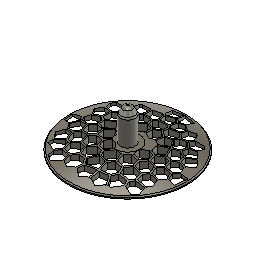
CD Labeler v6 (Autodesk Fusion 360 design; units mm, degrees)
Autodesk Fusion 360 part; units mm, degrees
sketch "Sketch1" plane through (0, 0, 0) normal (0, 0, 1) x (1, 0, 0)
  line L0 (0, 0) -> (-60, 0)
  line L1 (0, 40) -> (-7.4, 40)
  line L2 (-7.4, 40) -> (-7.4, 7.5)
  line L3 (-7.4, 7.5) -> (-12.4, 7.5)
  line L4 (-60, 0) -> (-60, 2)
  spline S0 degree 5 poles (-60, 2) (-58.1311, 2.342) (-54.3892, 3.0118) (-48.7641, 3.9741) (-41.2378, 5.166) (-31.765, 6.4302) (-24.1021, 7.147) (-18.2833, 7.4358) (-14.3673, 7.5) (-12.4, 7.5) knots 0 0 0 0 0 0 0.2 0.4 0.6 0.8 1 1 1 1 1 1
  line L5 (-17.4, 7.5) -> (-7.4, 7.5)
  line L6 (0, 40) -> (0, 0)
  dimension "d5" = 60
  dimension "d6" = 40
  dimension "d7" = 7.5
  dimension "d8" = 5
  dimension "d9" = 7.4
  dimension "d10" = 2
  constraint coincident L0.start L6.end
  constraint horizontal L0
  constraint perpendicular L1 L2
  constraint perpendicular L2 L3
  constraint vertical L0.start L1.start
  constraint perpendicular L0 L4
  constraint midpoint L3.end L5
  constraint coincident L2.end L3.start
  measures "d5" distance of L0.start L0.end
  measures "d6" distance of L0.start L1.start
  measures "d7" distance of L0 L3
  measures "d8" distance of L2.end L3.end
  measures "d9" distance of L0.start L2
  measures "d10" distance of L0.end L4.end
revolve "Revolve1" add sketch "Sketch1" angle 360 about axis through (0, 40, 0) along (0, -1, 0)
chamfer "Chamfer1" distance 4 angle 60 1 edges at (-6.8992, 40, 2.676) measured on face at (-1.4729, 40, 2.6203)
fillet "Fillet1" radius 4 2 edges at (-3.1699, 40, -1.2295) (-6.8992, 33.0718, 2.676)
chamfer "Chamfer2" distance 1 angle 45 1 edges at (-55.9396, 2, 21.6969) measured on face at (-50.8568, 3.2274, -15.1547)
sketch "Voronoi" plane through (0, 0, 0) normal (0, -1, 0) x (1, 0, 0)
  circle A0 centre (0, 0) radius 60
  line L0 (-27.9065, 13.1696) -> (-34.9281, 12.0421)
  line L1 (-34.9281, 12.0421) -> (-38.6848, 16.0627)
  line L2 (-38.6848, 16.0627) -> (-35.8746, 24.3668)
  line L3 (-35.8746, 24.3668) -> (-32.044, 25.7826)
  line L4 (-32.044, 25.7826) -> (-26.0586, 21.4152)
  line L5 (-26.0586, 21.4152) -> (-27.9065, 13.1696)
  line L6 (10.5368, 0.5792) -> (4.8128, -2.3641)
  line L7 (4.8128, -2.3641) -> (0.9891, -1.0588)
  line L8 (0.9891, -1.0588) -> (-2.1672, 4.4874)
  line L9 (-2.1672, 4.4874) -> (1.2988, 10.7375)
  line L10 (1.2988, 10.7375) -> (7.2211, 11.6685)
  line L11 (7.2211, 11.6685) -> (11.5672, 7.4823)
  line L12 (11.5672, 7.4823) -> (10.5368, 0.5792)
  line L13 (-35.0108, -24.4064) -> (-34.1777, -32.4462)
  line L14 (-34.1777, -32.4462) -> (-44.9989, -34.043)
  line L15 (-44.9989, -34.043) -> (-47.8212, -30.2156)
  line L16 (-47.8212, -30.2156) -> (-46.0411, -24.2468)
  line L17 (-46.0411, -24.2468) -> (-38.1193, -22.0129)
  line L18 (-38.1193, -22.0129) -> (-35.0108, -24.4064)
  line L19 (-19.5879, 24.2667) -> (-25.0625, 22.7039)
  line L20 (-25.0625, 22.7039) -> (-31.0479, 27.0713)
  line L21 (-31.0479, 27.0713) -> (-29.3019, 34.4485)
  line L22 (-29.3019, 34.4485) -> (-21.5865, 36.5994)
  line L23 (-21.5865, 36.5994) -> (-17.0949, 32.1475)
  line L24 (-17.0949, 32.1475) -> (-19.5879, 24.2667)
  line L25 (-46.2354, -10.1125) -> (-38.6533, -12.4637)
  line L26 (-38.6533, -12.4637) -> (-38.56, -20.628)
  line L27 (-38.56, -20.628) -> (-46.4818, -22.862)
  line L28 (-46.4818, -22.862) -> (-50.7842, -17.082)
  line L29 (-50.7842, -17.082) -> (-46.2354, -10.1125)
  line L30 (-8.096, -27.9757) -> (-9.18, -32.5512)
  line L31 (-9.18, -32.5512) -> (-18.5579, -34.2016)
  line L32 (-18.5579, -34.2016) -> (-20.6222, -32.1222)
  line L33 (-20.6222, -32.1222) -> (-19.5242, -22.5311)
  line L34 (-19.5242, -22.5311) -> (-13.2488, -21.94)
  line L35 (-13.2488, -21.94) -> (-8.096, -27.9757)
  line L36 (39.3425, 0.2337) -> (45.9107, 0.9874)
  line L37 (45.9107, 0.9874) -> (49.7447, -4.1853)
  line L38 (49.7447, -4.1853) -> (47.1146, -9.6574)
  line L39 (47.1146, -9.6574) -> (41.0309, -11.0528)
  line L40 (41.0309, -11.0528) -> (36.8887, -6.9194)
  line L41 (36.8887, -6.9194) -> (39.3425, 0.2337)
  line L42 (-18.027, -5.9471) -> (-24.1755, -13.3608)
  line L43 (-24.1755, -13.3608) -> (-32.371, -8.4307)
  line L44 (-32.371, -8.4307) -> (-31.6276, -3.0621)
  line L45 (-31.6276, -3.0621) -> (-24.5907, -0.2592)
  line L46 (-24.5907, -0.2592) -> (-18.027, -5.9471)
  line L47 (10.7696, 22.7391) -> (6.3027, 27.2437)
  line L48 (6.3027, 27.2437) -> (8.1302, 35.9137)
  line L49 (8.1302, 35.9137) -> (8.6268, 36.3055)
  line L50 (8.6268, 36.3055) -> (17.3076, 34.8942)
  line L51 (17.3076, 34.8942) -> (20.1346, 29.6995)
  line L52 (20.1346, 29.6995) -> (17.7876, 23.9489)
  line L53 (17.7876, 23.9489) -> (10.7696, 22.7391)
  line L54 (-11.0886, 4.3113) -> (-15.7382, -4.7739)
  line L55 (-15.7382, -4.7739) -> (-17.0875, -4.8798)
  line L56 (-17.0875, -4.8798) -> (-23.6512, 0.8081)
  line L57 (-23.6512, 0.8081) -> (-22.375, 7.5716)
  line L58 (-22.375, 7.5716) -> (-15.122, 9.0483)
  line L59 (-15.122, 9.0483) -> (-11.0886, 4.3113)
  line L60 (33.8324, -27.9238) -> (33.0464, -21.9044)
  line L61 (33.0464, -21.9044) -> (39.3933, -18.8795)
  line L62 (39.3933, -18.8795) -> (45.5831, -24.6473)
  line L63 (45.5831, -24.6473) -> (39.9794, -30.3799)
  line L64 (39.9794, -30.3799) -> (33.8324, -27.9238)
  line L65 (-6.1734, 20.3155) -> (-12.2476, 18.5647)
  line L66 (-12.2476, 18.5647) -> (-18.0321, 23.7761)
  line L67 (-18.0321, 23.7761) -> (-15.5391, 31.657)
  line L68 (-15.5391, 31.657) -> (-9.0862, 32.5632)
  line L69 (-9.0862, 32.5632) -> (-4.1809, 24.8404)
  line L70 (-4.1809, 24.8404) -> (-6.1734, 20.3155)
  line L71 (-9.34, 34.3958) -> (-15.793, 33.4895)
  line L72 (-15.793, 33.4895) -> (-20.2846, 37.9414)
  line L73 (-20.2846, 37.9414) -> (-19.1442, 45.1176)
  line L74 (-19.1442, 45.1176) -> (-13.5017, 48.1808)
  line L75 (-13.5017, 48.1808) -> (-7.4331, 45.104)
  line L76 (-7.4331, 45.104) -> (-6.1591, 39.3578)
  line L77 (-6.1591, 39.3578) -> (-9.34, 34.3958)
  line L78 (12.2231, 0.3468) -> (13.2535, 7.25)
  line L79 (13.2535, 7.25) -> (20.8866, 9.2558)
  line L80 (20.8866, 9.2558) -> (25.2818, 4.1153)
  line L81 (25.2818, 4.1153) -> (23.592, -1.8074)
  line L82 (23.592, -1.8074) -> (18.3034, -3.8239)
  line L83 (18.3034, -3.8239) -> (12.2231, 0.3468)
  line L84 (21.6213, 30.6504) -> (18.7944, 35.8452)
  line L85 (18.7944, 35.8452) -> (23.926, 44.059)
  line L86 (23.926, 44.059) -> (26.7774, 44.2439)
  line L87 (26.7774, 44.2439) -> (32.4218, 36.8622)
  line L88 (32.4218, 36.8622) -> (30.8724, 31.3991)
  line L89 (30.8724, 31.3991) -> (21.6213, 30.6504)
  line L90 (5.4069, -28.6869) -> (5.7475, -34.199)
  line L91 (5.7475, -34.199) -> (3.4929, -36.7027)
  line L92 (3.4929, -36.7027) -> (-5.3646, -36.1946)
  line L93 (-5.3646, -36.1946) -> (-7.566, -32.9035)
  line L94 (-7.566, -32.9035) -> (-6.482, -28.3281)
  line L95 (-6.482, -28.3281) -> (0.1282, -25.3112)
  line L96 (0.1282, -25.3112) -> (5.4069, -28.6869)
  line L97 (-19.9419, -35.5296) -> (-20.3626, -43.7583)
  line L98 (-20.3626, -43.7583) -> (-21.5377, -44.6998)
  line L99 (-21.5377, -44.6998) -> (-30.0108, -44.8241)
  line L100 (-30.0108, -44.8241) -> (-31.5242, -43.6638)
  line L101 (-31.5242, -43.6638) -> (-31.8434, -34.2746)
  line L102 (-31.8434, -34.2746) -> (-22.0062, -33.4501)
  line L103 (-22.0062, -33.4501) -> (-19.9419, -35.5296)
  line L104 (20.2503, -26.6016) -> (26.1962, -18.8729)
  line L105 (26.1962, -18.8729) -> (31.4796, -22.0469)
  line L106 (31.4796, -22.0469) -> (32.2655, -28.0663)
  line L107 (32.2655, -28.0663) -> (27.2411, -32.7623)
  line L108 (27.2411, -32.7623) -> (21.77, -31.0504)
  line L109 (21.77, -31.0504) -> (20.2503, -26.6016)
  line L110 (-8.9484, -12.5065) -> (-13.447, -20.2206)
  line L111 (-13.447, -20.2206) -> (-19.7224, -20.8116)
  line L112 (-19.7224, -20.8116) -> (-22.4798, -18.4615)
  line L113 (-22.4798, -18.4615) -> (-23.073, -14.1926)
  line L114 (-23.073, -14.1926) -> (-16.9244, -6.779)
  line L115 (-16.9244, -6.779) -> (-15.5751, -6.6731)
  line L116 (-15.5751, -6.6731) -> (-9.2991, -11.2456)
  line L117 (-9.2991, -11.2456) -> (-8.9484, -12.5065)
  line L118 (6.6615, 37.7021) -> (-4.4548, 39.7887)
  line L119 (-4.4548, 39.7887) -> (-5.7288, 45.5349)
  line L120 (-5.7288, 45.5349) -> (1.4543, 51.1494)
  line L121 (1.4543, 51.1494) -> (7.689, 46.826)
  line L122 (7.689, 46.826) -> (7.1581, 38.0939)
  line L123 (7.1581, 38.0939) -> (6.6615, 37.7021)
  line L124 (25.1249, -2.252) -> (26.8147, 3.6707)
  line L125 (26.8147, 3.6707) -> (34.0171, 5.2501)
  line L126 (34.0171, 5.2501) -> (37.9277, 0.7189)
  line L127 (37.9277, 0.7189) -> (35.4738, -6.4342)
  line L128 (35.4738, -6.4342) -> (30.5831, -7.2276)
  line L129 (30.5831, -7.2276) -> (25.1249, -2.252)
  line L130 (-6.7904, -37.2762) -> (-8.6269, -44.9673)
  line L131 (-8.6269, -44.9673) -> (-10.5349, -46.0558)
  line L132 (-10.5349, -46.0558) -> (-18.7903, -43.8643)
  line L133 (-18.7903, -43.8643) -> (-18.3696, -35.6356)
  line L134 (-18.3696, -35.6356) -> (-8.9918, -33.9851)
  line L135 (-8.9918, -33.9851) -> (-6.7904, -37.2762)
  line L136 (18.7449, -27.1831) -> (20.2646, -31.6319)
  line L137 (20.2646, -31.6319) -> (15.6531, -36.5554)
  line L138 (15.6531, -36.5554) -> (7.5022, -34.1578)
  line L139 (7.5022, -34.1578) -> (7.1615, -28.6457)
  line L140 (7.1615, -28.6457) -> (12.7, -24.7716)
  line L141 (12.7, -24.7716) -> (18.7449, -27.1831)
  line L142 (31.8493, 19.1103) -> (23.5487, 17.6337)
  line L143 (23.5487, 17.6337) -> (19.3824, 23.2491)
  line L144 (19.3824, 23.2491) -> (21.7294, 28.9997)
  line L145 (21.7294, 28.9997) -> (30.9805, 29.7483)
  line L146 (30.9805, 29.7483) -> (33.6345, 25.7523)
  line L147 (33.6345, 25.7523) -> (31.8493, 19.1103)
  line L148 (11.357, -0.8997) -> (17.4373, -5.0704)
  line L149 (17.4373, -5.0704) -> (16.2296, -11.9593)
  line L150 (16.2296, -11.9593) -> (11.6828, -14.4433)
  line L151 (11.6828, -14.4433) -> (7.185, -12.6772)
  line L152 (7.185, -12.6772) -> (5.633, -3.8429)
  line L153 (5.633, -3.8429) -> (11.357, -0.8997)
  line L154 (-46.7868, 1.4637) -> (-49.1351, -2.9212)
  line L155 (-49.1351, -2.9212) -> (-57.55, -2.0501)
  line L156 (-57.55, -2.0501) -> (-56.9638, 7.3301)
  line L157 (-56.9638, 7.3301) -> (-50.7559, 8.9572)
  line L158 (-50.7559, 8.9572) -> (-46.7868, 1.4637)
  line L159 (-15.4197, 10.7094) -> (-22.6726, 9.2326)
  line L160 (-22.6726, 9.2326) -> (-26.4039, 12.8113)
  line L161 (-26.4039, 12.8113) -> (-24.556, 21.0568)
  line L162 (-24.556, 21.0568) -> (-19.0813, 22.6196)
  line L163 (-19.0813, 22.6196) -> (-13.2968, 17.4081)
  line L164 (-13.2968, 17.4081) -> (-15.4197, 10.7094)
  line L165 (-3.6332, 3.5517) -> (-0.4769, -1.9945)
  line L166 (-0.4769, -1.9945) -> (-8.2798, -9.9739)
  line L167 (-8.2798, -9.9739) -> (-14.5557, -5.4015)
  line L168 (-14.5557, -5.4015) -> (-9.9061, 3.6837)
  line L169 (-9.9061, 3.6837) -> (-3.6332, 3.5517)
  line L170 (30.814, -8.8315) -> (35.7047, -8.0381)
  line L171 (35.7047, -8.0381) -> (39.8469, -12.1715)
  line L172 (39.8469, -12.1715) -> (38.6895, -17.6465)
  line L173 (38.6895, -17.6465) -> (32.3427, -20.6714)
  line L174 (32.3427, -20.6714) -> (27.0592, -17.4973)
  line L175 (27.0592, -17.4973) -> (27.0533, -17.4793)
  line L176 (27.0533, -17.4793) -> (30.814, -8.8315)
  line L177 (41.3929, -12.5451) -> (47.4767, -11.1498)
  line L178 (47.4767, -11.1498) -> (52.4317, -17.5736)
  line L179 (52.4317, -17.5736) -> (46.7772, -23.776)
  line L180 (46.7772, -23.776) -> (46.4254, -23.788)
  line L181 (46.4254, -23.788) -> (40.2355, -18.0202)
  line L182 (40.2355, -18.0202) -> (41.3929, -12.5451)
  line L183 (-5, 7) -> (-9.843, 5.505)
  line L184 (-9.843, 5.505) -> (-13.8764, 10.2421)
  line L185 (-13.8764, 10.2421) -> (-11.7536, 16.9409)
  line L186 (-11.7536, 16.9409) -> (-5.6795, 18.6918)
  line L187 (-5.6795, 18.6918) -> (-1, 12)
  line L188 (-1, 12) -> (-5, 7)
  line L189 (-22.0232, 38.2148) -> (-29.7386, 36.0638)
  line L190 (-29.7386, 36.0638) -> (-34.5387, 40.8032)
  line L191 (-34.5387, 40.8032) -> (-34.0534, 46.3134)
  line L192 (-34.0534, 46.3134) -> (-28.3874, 50.1625)
  line L193 (-28.3874, 50.1625) -> (-20.8829, 45.3909)
  line L194 (-20.8829, 45.3909) -> (-22.0232, 38.2148)
  line L195 (-40.0469, 16.507) -> (-46.5087, 16.0762)
  line L196 (-46.5087, 16.0762) -> (-50.209, 23.0919)
  line L197 (-50.209, 23.0919) -> (-45.0738, 29.1532)
  line L198 (-45.0738, 29.1532) -> (-37.2368, 24.8111)
  line L199 (-37.2368, 24.8111) -> (-40.0469, 16.507)
  line L200 (3.4152, -38.1517) -> (4.165, -45.5593)
  line L201 (4.165, -45.5593) -> (0.0358, -48.5203)
  line L202 (0.0358, -48.5203) -> (-7.2789, -45.3347)
  line L203 (-7.2789, -45.3347) -> (-5.4424, -37.6436)
  line L204 (-5.4424, -37.6436) -> (3.4152, -38.1517)
  line L205 (22.0947, 10.2973) -> (23.826, 16.1583)
  line L206 (23.826, 16.1583) -> (32.1267, 17.6349)
  line L207 (32.1267, 17.6349) -> (35.5448, 13.1881)
  line L208 (35.5448, 13.1881) -> (33.6924, 6.7363)
  line L209 (33.6924, 6.7363) -> (26.4899, 5.1569)
  line L210 (26.4899, 5.1569) -> (22.0947, 10.2973)
  line L211 (47.0478, 1.9135) -> (49.747, 8.3061)
  line L212 (49.747, 8.3061) -> (56.4783, 9.0889)
  line L213 (56.4783, 9.0889) -> (57.6508, -3.2227)
  line L214 (57.6508, -3.2227) -> (50.8818, -3.2592)
  line L215 (50.8818, -3.2592) -> (47.0478, 1.9135)
  line L216 (-25.2097, 1.1481) -> (-32.2465, -1.6548)
  line L217 (-32.2465, -1.6548) -> (-36.7808, 3.0476)
  line L218 (-36.7808, 3.0476) -> (-34.6863, 10.3627)
  line L219 (-34.6863, 10.3627) -> (-27.6647, 11.4903)
  line L220 (-27.6647, 11.4903) -> (-23.9334, 7.9116)
  line L221 (-23.9334, 7.9116) -> (-25.2097, 1.1481)
  line L222 (-32.7309, 27.4491) -> (-36.5616, 26.0333)
  line L223 (-36.5616, 26.0333) -> (-44.3986, 30.3754)
  line L224 (-44.3986, 30.3754) -> (-45.2076, 35.5094)
  line L225 (-45.2076, 35.5094) -> (-35.785, 39.5656)
  line L226 (-35.785, 39.5656) -> (-30.9849, 34.8262)
  line L227 (-30.9849, 34.8262) -> (-32.7309, 27.4491)
  line L228 (21.3355, -32.6788) -> (26.8067, -34.3907)
  line L229 (26.8067, -34.3907) -> (28.5514, -39.12)
  line L230 (28.5514, -39.12) -> (25.3697, -45.2514)
  line L231 (25.3697, -45.2514) -> (23.23, -46.0964)
  line L232 (23.23, -46.0964) -> (17.8051, -43.7932)
  line L233 (17.8051, -43.7932) -> (16.724, -37.6022)
  line L234 (16.724, -37.6022) -> (21.3355, -32.6788)
  line L235 (22.7548, 44.773) -> (17.6232, 36.5592)
  line L236 (17.6232, 36.5592) -> (8.9424, 37.9705)
  line L237 (8.9424, 37.9705) -> (9.4732, 46.7025)
  line L238 (9.4732, 46.7025) -> (16.5801, 50.2354)
  line L239 (16.5801, 50.2354) -> (22.7548, 44.773)
  line L240 (17.6848, -12.2585) -> (18.8925, -5.3696)
  line L241 (18.8925, -5.3696) -> (24.1811, -3.3531)
  line L242 (24.1811, -3.3531) -> (29.6394, -8.3287)
  line L243 (29.6394, -8.3287) -> (25.8788, -16.9765)
  line L244 (25.8788, -16.9765) -> (17.6848, -12.2585)
  line L245 (-34.2135, -8.1609) -> (-38.159, -11.0326)
  line L246 (-38.159, -11.0326) -> (-45.7412, -8.6814)
  line L247 (-45.7412, -8.6814) -> (-47.6362, -3.8307)
  line L248 (-47.6362, -3.8307) -> (-45.2879, 0.5542)
  line L249 (-45.2879, 0.5542) -> (-38.0043, 1.9101)
  line L250 (-38.0043, 1.9101) -> (-33.4701, -2.7923)
  line L251 (-33.4701, -2.7923) -> (-34.2135, -8.1609)
  line L252 (-21.0665, -22.3256) -> (-22.1644, -31.9167)
  line L253 (-22.1644, -31.9167) -> (-32.0016, -32.7411)
  line L254 (-32.0016, -32.7411) -> (-32.5231, -32.2458)
  line L255 (-32.5231, -32.2458) -> (-33.3562, -24.2061)
  line L256 (-33.3562, -24.2061) -> (-23.8239, -19.9754)
  line L257 (-23.8239, -19.9754) -> (-21.0665, -22.3256)
  line L258 (-38.2811, 3.473) -> (-45.5647, 2.1171)
  line L259 (-45.5647, 2.1171) -> (-49.5338, 9.6106)
  line L260 (-49.5338, 9.6106) -> (-46.4051, 14.378)
  line L261 (-46.4051, 14.378) -> (-39.9434, 14.8088)
  line L262 (-39.9434, 14.8088) -> (-36.1867, 10.7882)
  line L263 (-36.1867, 10.7882) -> (-38.2811, 3.473)
  line L264 (9.4794, 21.5065) -> (6.9532, 13.4202)
  line L265 (6.9532, 13.4202) -> (1.0309, 12.4892)
  line L266 (1.0309, 12.4892) -> (-4.5446, 19.5579)
  line L267 (-4.5446, 19.5579) -> (-2.552, 24.0828)
  line L268 (-2.552, 24.0828) -> (5.0126, 26.011)
  line L269 (5.0126, 26.011) -> (9.4794, 21.5065)
  line L270 (11.0684, -16.0265) -> (11.8244, -23.5958)
  line L271 (11.8244, -23.5958) -> (6.2859, -27.4699)
  line L272 (6.2859, -27.4699) -> (1.0072, -24.0942)
  line L273 (1.0072, -24.0942) -> (1.1658, -17.3926)
  line L274 (1.1658, -17.3926) -> (6.5707, -14.2604)
  line L275 (6.5707, -14.2604) -> (11.0684, -16.0265)
  line L276 (-2.9306, 25.6066) -> (-7.8358, 33.3294)
  line L277 (-7.8358, 33.3294) -> (-4.6549, 38.2914)
  line L278 (-4.6549, 38.2914) -> (6.4615, 36.2049)
  line L279 (6.4615, 36.2049) -> (4.634, 27.5349)
  line L280 (4.634, 27.5349) -> (-2.9306, 25.6066)
  line L281 (32.5436, 30.8768) -> (34.0929, 36.3399)
  line L282 (34.0929, 36.3399) -> (42.7798, 39.3092)
  line L283 (42.7798, 39.3092) -> (46.5254, 34.4849)
  line L284 (46.5254, 34.4849) -> (44.5268, 27.3885)
  line L285 (44.5268, 27.3885) -> (35.1977, 26.8808)
  line L286 (35.1977, 26.8808) -> (32.5436, 30.8768)
  line L287 (-10, -55) -> (-9.6654, -47.4752)
  line L288 (-9.6654, -47.4752) -> (-7.7574, -46.3868)
  line L289 (-7.7574, -46.3868) -> (-0.4427, -49.5724)
  line L290 (-0.4427, -49.5724) -> (-0.4939, -57.3118)
  line L291 (-0.4939, -57.3118) -> (-10, -55)
  line L292 (5.0928, -46.6266) -> (10.714, -48.7836)
  line L293 (10.714, -48.7836) -> (12.2154, -55.4002)
  line L294 (12.2154, -55.4002) -> (0.9125, -57.3271)
  line L295 (0.9125, -57.3271) -> (0.9637, -49.5877)
  line L296 (0.9637, -49.5877) -> (5.0928, -46.6266)
  line L297 (33.2399, -29.1078) -> (39.387, -31.5638)
  line L298 (39.387, -31.5638) -> (40.5405, -36.8524)
  line L299 (40.5405, -36.8524) -> (37.9065, -39.8846)
  line L300 (37.9065, -39.8846) -> (29.9603, -38.5331)
  line L301 (29.9603, -38.5331) -> (28.2155, -33.8038)
  line L302 (28.2155, -33.8038) -> (33.2399, -29.1078)
  line L303 (4.1413, -4.0477) -> (5.6933, -12.882)
  line L304 (5.6933, -12.882) -> (0.2884, -16.0141)
  line L305 (0.2884, -16.0141) -> (-7.1347, -11.9828)
  line L306 (-7.1347, -11.9828) -> (-7.4854, -10.7219)
  line L307 (-7.4854, -10.7219) -> (-4, -7)
  line L308 (-4, -7) -> (4.1413, -4.0477)
  line L309 (15.2819, -37.8547) -> (16.363, -44.0456)
  line L310 (16.363, -44.0456) -> (11.2473, -47.5253)
  line L311 (11.2473, -47.5253) -> (5.6261, -45.3684)
  line L312 (5.6261, -45.3684) -> (4.8764, -37.9609)
  line L313 (4.8764, -37.9609) -> (7.131, -35.4571)
  line L314 (7.131, -35.4571) -> (15.2819, -37.8547)
  line L315 (20.4789, 10.7933) -> (12.8458, 8.7875)
  line L316 (12.8458, 8.7875) -> (8.4997, 12.9736)
  line L317 (8.4997, 12.9736) -> (11.0259, 21.0599)
  line L318 (11.0259, 21.0599) -> (18.044, 22.2696)
  line L319 (18.044, 22.2696) -> (22.2103, 16.6542)
  line L320 (22.2103, 16.6542) -> (20.4789, 10.7933)
  line L321 (-0.363, -17.3068) -> (-0.5216, -24.0084)
  line L322 (-0.5216, -24.0084) -> (-7.1318, -27.0253)
  line L323 (-7.1318, -27.0253) -> (-12.2846, -20.9895)
  line L324 (-12.2846, -20.9895) -> (-7.786, -13.2755)
  line L325 (-7.786, -13.2755) -> (-0.363, -17.3068)
  line L326 (17.1188, -13.3939) -> (25.3128, -18.1119)
  line L327 (25.3128, -18.1119) -> (25.3187, -18.1299)
  line L328 (25.3187, -18.1299) -> (19.3728, -25.8587)
  line L329 (19.3728, -25.8587) -> (13.3279, -23.4471)
  line L330 (13.3279, -23.4471) -> (12.572, -15.8778)
  line L331 (12.572, -15.8778) -> (17.1188, -13.3939)
  line L332 (33.5158, 18.67) -> (35.301, 25.312)
  line L333 (35.301, 25.312) -> (44.6302, 25.8197)
  line L334 (44.6302, 25.8197) -> (47.2763, 21.8917)
  line L335 (47.2763, 21.8917) -> (44.9202, 15.1471)
  line L336 (44.9202, 15.1471) -> (36.934, 14.2232)
  line L337 (36.934, 14.2232) -> (33.5158, 18.67)
  line L338 (-33.0188, -9.5674) -> (-24.8233, -14.4974)
  line L339 (-24.8233, -14.4974) -> (-24.2302, -18.7663)
  line L340 (-24.2302, -18.7663) -> (-33.7625, -22.997)
  line L341 (-33.7625, -22.997) -> (-36.8711, -20.6034)
  line L342 (-36.8711, -20.6034) -> (-36.9643, -12.4391)
  line L343 (-36.9643, -12.4391) -> (-33.0188, -9.5674)
  line L344 (39.1658, 1.7636) -> (35.2553, 6.2948)
  line L345 (35.2553, 6.2948) -> (37.1078, 12.7467)
  line L346 (37.1078, 12.7467) -> (45.094, 13.6706)
  line L347 (45.094, 13.6706) -> (48.4332, 8.9099)
  line L348 (48.4332, 8.9099) -> (45.734, 2.5174)
  line L349 (45.734, 2.5174) -> (39.1658, 1.7636)
extrude "Extrude2" cut sketch "Voronoi" against normal through all contours L0 L1 L2 L3 L4 L5 | L13 L14 L15 L16 L17 L18 | L19 L20 L21 L22 L23 L24 | L25 L26 L27 L28 L29 | L30 L31 L32 L33 L34 L35 | L36 L37 L38 L39 L40 L41 | L42 L43 L44 L45 L46 | L47 L48 L49 L50 L51 L52 L53 | L54 L55 L56 L57 L58 L59 | L60 L61 L62 L63 L64 | L65 L66 L67 L68 L69 L70 | L71 L72 L73 L74 L75 L76 L77 | L78 L79 L80 L81 L82 L83 | L84 L85 L86 L87 L88 L89 | L90 L91 L92 L93 L94 L95 L96 | L97 L98 L99 L100 L101 L102 L103 | L104 L105 L106 L107 L108 L109 | L110 L111 L112 L113 L114 L115 L116 L117 | L118 L119 L120 L121 L122 L123 | L124 L125 L126 L127 L128 L129 | L130 L131 L132 L133 L134 L135 | L136 L137 L138 L139 L140 L141 | L142 L143 L144 L145 L146 L147 | L154 L155 L156 L157 L158 | L159 L160 L161 L162 L163 L164 | L170 L171 L172 L173 L174 L175 L176 | L177 L178 L179 L180 L181 L182 | L183 L184 L185 L186 L187 L188 | L189 L190 L191 L192 L193 L194 | L195 L196 L197 L198 L199 | L200 L201 L202 L203 L204 | L205 L206 L207 L208 L209 L210 | L211 L212 L213 L214 L215 | L216 L217 L218 L219 L220 L221 | L222 L223 L224 L225 L226 L227 | L228 L229 L230 L231 L232 L233 L234 | L235 L236 L237 L238 L239 | L240 L241 L242 L243 L244 | L245 L246 L247 L248 L249 L250 L251 | L252 L253 L254 L255 L256 L257 | L258 L259 L260 L261 L262 L263 | L264 L265 L266 L267 L268 L269 | L270 L271 L272 L273 L274 L275 | L276 L277 L278 L279 L280 | L281 L282 L283 L284 L285 L286 | L287 L288 L289 L290 L291 | L292 L293 L294 L295 L296 | L297 L298 L299 L300 L301 L302 | L309 L310 L311 L312 L313 L314 | L315 L316 L317 L318 L319 L320 | L321 L322 L323 L324 L325 | L326 L327 L328 L329 L330 L331 | L332 L333 L334 L335 L336 L337 | L338 L339 L340 L341 L342 L343 | L344 L345 L346 L347 L348 L349
equation "d5 = ( 120 / 2 ) * 1 mm"
equation "d9 = ( 14.8 / 2 ) * 1 mm"
named bodies: "CdLabeler"
